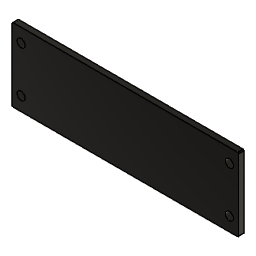
Galaxy_rear_panel (Autodesk Fusion 360 design; units mm, degrees)
Autodesk Fusion 360 part; units mm, degrees
sketch "Sketch1" plane through (0, 0, 0) normal (0, 1, 0) x (1, 0, 0)
  line L0 (-61.5, -20) -> (61.5, -20)
  line L1 (62, -19.5) -> (62, 19.5)
  line L2 (61.5, 20) -> (-61.5, 20)
  line L3 (-62, 19.5) -> (-62, -19.5)
  line L4 (-62, -20) -> (62, 20) construction
  line L5 (62, -20) -> (-62, 20) construction
  line L6 (62, 20) -> (57, 20)
  line L7 (57, 20) -> (57, 12.5) construction
  line L8 (57, 12.5) -> (62, 12.5) construction
  line L9 (62, 12.5) -> (62, 20)
  line L10 (62, -20) -> (57, -20)
  line L11 (57, -20) -> (57, -12.5) construction
  line L12 (57, -12.5) -> (62, -12.5) construction
  line L13 (62, -12.5) -> (62, -20)
  line L14 (-62, -20) -> (-57, -20)
  line L15 (-57, -20) -> (-57, -12.5) construction
  line L16 (-57, -12.5) -> (-62, -12.5) construction
  line L17 (-62, -12.5) -> (-62, -20)
  line L18 (-62, 20) -> (-57, 20)
  line L19 (-57, 20) -> (-57, 12.5) construction
  line L20 (-57, 12.5) -> (-62, 12.5) construction
  line L21 (-62, 12.5) -> (-62, 20)
  circle A0 centre (57, -12.5) radius 2.2
  circle A1 centre (-57, -12.5) radius 2.2
  circle A2 centre (57, 12.5) radius 2.2
  circle A3 centre (-57, 12.5) radius 2.2
  arc A4 (61.5, -20) -> (62, -19.5) centre (61.5, -19.5) ccw
  arc A5 (-62, -19.5) -> (-61.5, -20) centre (-61.5, -19.5) ccw
  arc A6 (-61.5, 20) -> (-62, 19.5) centre (-61.5, 19.5) ccw
  arc A7 (62, 19.5) -> (61.5, 20) centre (61.5, 19.5) ccw
  dimension "d1" = 124
  dimension "d2" = 40
  dimension "d3" = 5
  dimension "d4" = 7.5
  dimension "d5" = 5
  dimension "d6" = 7.5
  dimension "d7" = 5
  dimension "d8" = 7.5
  dimension "d9" = 5
  dimension "d10" = 7.5
  dimension "d11" = 4.4
  dimension "d12" = 4.4
  dimension "d13" = 4.4
  dimension "d14" = 4.4
  dimension "d15" = 0.5
  constraint horizontal L0
  constraint perpendicular L0 L1
  constraint parallel L0 L2
  constraint parallel L1 L3
  constraint coincident L4 origin
  constraint coincident L5 origin
  constraint horizontal L6
  constraint vertical L7
  constraint horizontal L8
  constraint vertical L9
  constraint horizontal L10
  constraint vertical L11
  constraint horizontal L12
  constraint vertical L13
  constraint horizontal L14
  constraint vertical L15
  constraint horizontal L16
  constraint vertical L17
  constraint horizontal L18
  constraint vertical L19
  constraint horizontal L20
  constraint vertical L21
  constraint coincident L11.end L12.start
  constraint coincident L15.end L16.start
  constraint coincident L7.end L8.start
  constraint coincident L19.end L20.start
  constraint coincident L5.start L1
  constraint coincident L5.start L0
  constraint tangent L1 A4
  constraint tangent L0 A4
  constraint coincident L4.start L0
  constraint coincident L4.start L3
  constraint tangent L0 A5
  constraint tangent L3 A5
  constraint equal A4 A5
  constraint coincident L5.end L3
  constraint coincident L5.end L2
  constraint tangent L3 A6
  constraint tangent L2 A6
  constraint equal A4 A6
  constraint coincident L4.end L2
  constraint coincident L4.end L1
  constraint tangent L2 A7
  constraint tangent L1 A7
  constraint equal A4 A7
  measures "d1" distance of L4.end L5.end
  measures "d2" distance of L5.start L4.end
  measures "d3" distance of L4.end L6.end
  measures "d4" distance of L4.end L8.end
  measures "d5" distance of L5.start L10.end
  measures "d6" distance of L5.start L12.end
  measures "d7" distance of L4.start L14.end
  measures "d8" distance of L4.start L16.end
  measures "d9" distance of L5.end L18.end
  measures "d10" distance of L5.end L20.end
  measures "d11" diameter of A0
  measures "d12" diameter of A1
  measures "d13" diameter of A2
  measures "d14" diameter of A3
  measures "d15" radius of A4
extrude "Extrude1" add sketch "Sketch1" along normal blind 3 contours L0 L1 L2 L3 L6 L9 L10 L13 L14 L17 L18 L21 A4 A5 A6 A7
